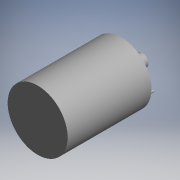
# Autodesk Inventor part: motor_body
Saved by Autodesk Inventor 2019.4 (Build 234330000, 330)
## iProperties
Created: 2020-06-20
Part Number: motor_body
Material: Generic
Document SubType Name: Modeling
Designer: Jorge
Density: 1 g/cm^3
Appearance: Default
Author: Jorge
Autodesk Inventor part; units mm, degrees
ref_plane "YZ Plane" through (0, 0, 0) normal (1, 0, 0) x (0, 1, 0)
ref_plane "XZ Plane" through (0, 0, 0) normal (0, 1, 0) x (-1, 0, 0)
ref_plane "XY Plane" through (0, 0, 0) normal (0, 0, 1) x (1, 0, 0)
sketch "Sketch1" plane through (0, 0, 0) normal (0, 0, 1) x (1, 0, 0)
  circle A0 centre (0, 0) radius 12.2
  dimension "d0" = 24.4
  constraints: 1 centre point, 1 coincident
  measures "d0" diameter of A0
extrude "Extrusion1" add sketch "Sketch1" along normal blind 34
sketch "Sketch2" plane through (0, 0, 0) normal (0, 0, -1) x (-1, 0, 0)
  circle A0 centre (0, 0) radius 2.5
  dimension "d3" = 5
  constraints: 1 centre point, 1 coincident
  measures "d3" diameter of A0
extrude "Extrusion2" add sketch "Sketch2" along normal blind 8.5
sketch "Sketch3" plane through (0, 0, 0) normal (0, 0, -1) x (-1, 0, 0)
  line L0 (-3.25, -8) -> (3.25, -8) construction
  line L1 (3.25, -8) -> (3.25, -10.5) construction
  line L2 (3.25, -10.5) -> (-3.25, -10.5) construction
  line L3 (-3.25, -10.5) -> (-3.25, -8) construction
  line L4 (0, 0) -> (-3.25, -8) construction
  line L5 (3.25, -8) -> (0, 0) construction
  line L6 (0, 0) -> (0, -8) construction
  line L7 (-7.955, -3.3588) -> (-3.3588, -7.955) construction
  line L8 (-3.3588, -7.955) -> (-5.1265, -9.7227) construction
  line L9 (-5.1265, -9.7227) -> (-9.7227, -5.1265) construction
  line L10 (-9.7227, -5.1265) -> (-7.955, -3.3588) construction
  line L11 (0, 0) -> (-7.955, -3.3588) construction
  line L12 (-3.3588, -7.955) -> (0, 0) construction
  line L13 (0, 0) -> (-5.6569, -5.6569) construction
  circle A0 centre (-2.0637, -9.25) radius 0.5
  circle A1 centre (2.0568, -9.25) radius 0.5
  circle A2 centre (0, -9.25) radius 0.5
  circle A3 centre (-6.5905, -6.5905) radius 0.5
  circle A4 centre (-5.1265, -7.955) radius 0.5
  circle A5 centre (-7.9716, -5.1098) radius 0.5
  dimension "d6" = 2.5
  dimension "d7" = 6.5
  dimension "d8" = 8
  dimension "d9" = 2.5
  dimension "d10" = 6.5
  dimension "d11" = 8
  dimension "d12" = 45
  dimension "d13" = 1
  dimension "d14" = 1
  dimension "d15" = 1
  dimension "d18" = 1
  dimension "d19" = 1
  dimension "d20" = 1
  constraints: 30 end point, 6 centre point, 6 perpendicular, 2 equal length, 2 midpoint, 1 vertical
  measures "d6" distance of L0.end L1.end
  measures "d7" distance of L1.end L2.end
  measures "d8" distance of L4.start L6.end
  measures "d9" distance of L7.end L8.end
  measures "d10" distance of L8.end L9.end
  measures "d11" distance of L4.start L13.end
  measures "d12" angle of L13 L6
  measures "d13" diameter of A0
  measures "d14" diameter of A1
  measures "d15" diameter of A2
  measures "d18" diameter of A3
  measures "d19" diameter of A4
  measures "d20" diameter of A5
extrude "Extrusion3" add sketch "Sketch3" along normal blind 5 contours A0 | A1 | A2
extrude "Extrusion4" add sketch "Sketch3" along normal blind 5 contours A3 | A4 | A5
body "Solid1"
